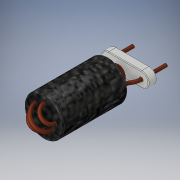
# Autodesk Inventor part: LairdTech_28C0236-0JW-10__
Saved by Autodesk Inventor 2019.1 (Build 231200000, 200)
## iProperties
Created: 2018-10-28
Part Number: LairdTech_28C0236-0JW-10__
Material: Generic
Document SubType Name: Modeling
Designer: huesof
Density: 1 g/cm^3
Appearance: Default
Author: huesof
Autodesk Inventor part; units mm, degrees
ref_plane "YZ Plane" through (0, 0, 0) normal (1, 0, 0) x (0, 1, 0)
ref_plane "XZ Plane" through (0, 0, 0) normal (0, 1, 0) x (-1, 0, 0)
ref_plane "XY Plane" through (0, 0, 0) normal (0, 0, 1) x (1, 0, 0)
sketch "Sketch1" plane through (0, 0, 0) normal (0, 0, 1) x (1, 0, 0)
  circle A0 centre (0, 0) radius 1.143
  circle A1 centre (5.08, 0) radius 1.143
  line L0 (0, 0) -> (0, 1.143) construction
  line L1 (5.08, 0) -> (5.08, 1.143) construction
  line L2 (0, 0) -> (0, -1.143) construction
  line L3 (5.08, 0) -> (5.08, -1.143) construction
  line L4 (0, 1.143) -> (5.08, 1.143)
  line L5 (5.08, -1.143) -> (0, -1.143)
  circle A2 centre (0, 0) radius 0.254
  circle A3 centre (5.08, 0) radius 0.254
  point P0 (1.7349, 0.2538)
  dimension "d0" = 2.286
  dimension "d1" = 2.286
  dimension "d2" = 0
  dimension "d3" = 5.08
  dimension "d4" = 0.508
  dimension "d5" = 0.508
  constraints: 12 end point, 5 coincident, 4 centre point, 4 point on circle, 2 point on line, 2 tangent, 1 parallel, 1 perpendicular
  measures "d0" diameter of A0
  measures "d1" diameter of A1
  measures "d2" vertical distance of point (0, 0) A1.centre
  measures "d3" distance of A1.centre point (0, 0)
  measures "d4" diameter of A2
  measures "d5" diameter of A3
extrude "Extrusion1" add sketch "Sketch1" along normal blind 1.27 contours A0 | A0 L4 A1 L5 | A1 | A2 | A3
hole "Hole1" at (5.08, 0, 0) at (0, 0, 0) direction (0, 0, 1) diameter 0.635 depth 1.27
extrude "Extrusion2" add sketch "Sketch1" along normal up to surface (1.27 mm away) separate body contours A2 | A3
extrude "Extrusion3" add sketch "Sketch1" against normal blind 5.08 contours A2 | A3 bodies 2
ref_plane "Work Plane1" through (0, 0, 3.81) normal (0, 0, 1) x (1, 0, 0)
sketch "Sketch2" plane through (0, 0, 3.81) normal (0, 0, 1) x (1, 0, 0)
  circle A0 centre (5.08, 0) radius 0.254 projected
  circle A1 centre (0, 0) radius 0.254 projected
  line L0 (0, 0) -> (5.08, 0) construction
  circle A2 centre (2.54, 0) radius 3
  circle A3 centre (2.54, 1.7526) radius 0.3175
  circle A4 centre (1.3007, 1.2393) radius 0.3175
  line L1 (2.54, 0) -> (1.3007, 1.2393) construction
  line L2 (2.54, 0) -> (4.2926, 0) construction
  circle A5 centre (0.7874, 0) radius 0.3175
  circle A6 centre (2.54, -1.7526) radius 0.3175
  circle A7 centre (3.7793, -1.2393) radius 0.3175
  circle A8 centre (4.2926, 0) radius 0.3175
  dimension "d20" = 6
  dimension "d24" = 0
  dimension "d26" = 1.7526
  dimension "d27" = 0.635
  dimension "d29" = 0.635
  dimension "d30" = 1.7526
  dimension "d31" = 225
  dimension "d36" = 0.635
  dimension "d37" = 1.7526
  dimension "d40" = 360
  constraints: 7 centre point, 6 end point, 2 coincident, 2 horizontal, 1 equal length, 1 midpoint, 1 point on line, 13 other
  measures "d20" diameter of A2
  measures "d24" horizontal distance of point (2.54, 0) A3.centre
  measures "d26" distance of point (2.54, 0) A3.centre
  measures "d27" diameter of A3
  measures "d29" diameter of A4
  measures "d30" distance of L1.start L1.end
  measures "d36" diameter of A5
  measures "d37" distance of point (2.54, 0) A5.centre
extrude "Extrusion4" add sketch "Sketch2" along normal blind 10 separate body contours A0 | A1 | A2
sketch "Sketch3" plane through (0, 0, 0) normal (0, 1, 0) x (-1, 0, 0)
  line L0 (-0.4699, 3.81) -> (-1.1049, 3.81) construction
  line L1 (-0.7874, 3.81) -> (0, 1.27) construction
  line L2 (-0.3175, 1.27) -> (0.3175, 1.27) construction
  line L3 (-5.3975, 1.27) -> (-4.7625, 1.27) construction
  line L4 (-5.08, 1.27) -> (-4.2926, 3.81) construction
  line L5 (-3.9751, 3.81) -> (-4.6101, 3.81) construction
  line L6 (0, 1.27) -> (-5.08, 1.27) construction
  arc A0 (-4.6863, 2.54) -> (-5.08, 1.27) centre (-2.5416, 1.1791) ccw
  line L7 (1.143, 1.27) -> (0, 1.27) projected
  arc A1 (0, 1.27) -> (-0.3937, 2.54) centre (-2.5384, 1.1791) ccw
  arc A2 (-0.7874, 3.81) -> (-0.3937, 2.54) centre (1.751, 3.9009) ccw
  arc A3 (-4.6863, 2.54) -> (-4.2926, 3.81) centre (-6.831, 3.9009) ccw
  point P0 (0, 0)
  dimension "d42" = 2.54
  dimension "d43" = 2.54
  dimension "d44" = 2.54
  dimension "d45" = 2.54
  constraints: 8 point on circle, 6 midpoint, 4 centre point, 4 end point, 2 point on line
  measures "d42" radius of A0
  measures "d43" radius of A1
  measures "d44" radius of A3
  measures "d45" radius of A2
sketch "Sketch4" plane through (5.08, 0, 1.27) normal (0, 0, 1) x (1, 0, 0)
  circle A0 centre (0, 0) radius 0.254 projected
  circle A1 centre (-5.08, 0) radius 0.254 projected
sweep "Sweep1" add profiles "Sketch4" path "Sketch3" bodies 2 path curves A0 A3 contours A0
sweep "Sweep2" add profiles "Sketch4" path "Sketch3" bodies 2 path curves A1 A2 contours A1
sketch "Sketch5" plane through (4.2926, 0, 3.81) normal (0, 0, 1) x (1, 0, 0)
  circle A0 centre (0, 0) radius 0.254 projected
  circle A1 centre (-3.5052, 0) radius 0.254 projected
  point P0 (-4.2926, 0)
  point P1 (0.254, 0)
  point P2 (-3.2512, 0)
  constraints: 2 horizontal alignment
extrude "Extrusion5" add sketch "Sketch5" along normal up to surface (10 mm away) bodies 2
sketch "Sketch6" plane through (0.7874, 0, 13.81) normal (0, 0, 1) x (1, 0, 0)
  circle A0 centre (0, 0) radius 0.254 projected
  circle A1 centre (3.5052, 0) radius 0.254 projected
  circle A2 centre (1.7526, 1.7526) radius 0.3175 projected
  circle A3 centre (0.5133, 1.2393) radius 0.3175 projected
  circle A4 centre (1.7526, -1.7526) radius 0.3175 projected
  circle A5 centre (2.9919, -1.2393) radius 0.3175 projected
  circle A6 centre (2.9919, -1.2393) radius 0.254
  line L0 (0, 0) -> (3.5052, 0) construction
  line L1 (1.7526, 0) -> (3.8739, 2.1213) construction
  line L2 (1.7526, 0) -> (4.7526, 0) construction
  circle A7 centre (1.7526, -1.7526) radius 0.254
  circle A8 centre (0.5133, 1.2393) radius 0.254
  circle A9 centre (1.7526, 1.7526) radius 0.254
  point P0 (-0.7874, 0)
  dimension "d52" = 0.508
  dimension "d53" = 0.508
  dimension "d54" = 3
  dimension "d55" = 45
  dimension "d57" = 0.508
  dimension "d59" = 0.508
  dimension "d61" = 0.508
  constraints: 6 end point, 4 centre point, 4 coincident, 2 horizontal, 1 equal length, 1 midpoint
  measures "d52" diameter of A6
  measures "d53" diameter of A1
  measures "d54" distance of L1.start L1.end
  measures "d55" angle of L2 L1
  measures "d57" diameter of A7
  measures "d59" diameter of A8
  measures "d61" diameter of A9
revolve "Revolution1" add sketch "Sketch6" angle 180 about axis through (2.54, 0, 13.81) along (-0.7071068, -0.7071068, 0) bodies 2 contours A1 | A6 | A7
extrude "Extrusion6" add sketch "Sketch6" against normal up to surface (10 mm away) contours A6 | A7 | A8 | A9 bodies 2
sketch "Sketch7" plane through (2.54, -1.7526, 3.81) normal (0, 0, -1) x (-1, 0, 0)
  circle A0 centre (0, 0) radius 0.254 projected
  circle A1 centre (-1.2393, 0.5133) radius 0.254 projected
  circle A2 centre (1.2393, 2.9919) radius 0.254 projected
  circle A3 centre (0, 3.5052) radius 0.254 projected
  circle A4 centre (-1.2393, 0.5133) radius 0.3175 construction
  line L0 (-1.2393, 0.5133) -> (1.2393, 2.9919) construction
  line L1 (0, 0) -> (0, 3.5052) construction
  line L2 (0, 1.7526) -> (-0.8423, 2.1015) construction
  line L3 (1.2393, 2.9919) -> (0, 3.5052) construction
  point P0 (2.54, 1.7526)
  constraints: 8 end point, 1 midpoint, 1 parallel, 1 vertical
revolve "Revolution2" add sketch "Sketch7" angle 180 about axis through (2.54, 0, 3.81) along (0.9238795, 0.3826834, 0) bodies 2 contours A0 | A1
fillet "Fillet1" radius 0.2 2 edges at (-0.46, 0, 13.81) (-0.46, 0, 3.81)
fillet "Fillet2" radius 0.1 8 edges at (-1.143, 0, 1.27) (2.54, -1.143, 1.27) (6.223, 0, 1.27) (2.54, 1.143, 1.27) (-1.143, 0, 0) (2.54, -1.143, 0) (6.223, 0, 0) (2.54, 1.143, 0)
thicken "Thicken1" operation add thickness 2.54 both sides no extend neighbours yes toward (0, 0, 1) bodies 2 faces at (-0.075, -0.0393, -5.08)
thicken "Thicken2" operation add thickness 2.54 both sides no extend neighbours yes toward (0, 0, 1) bodies 2 faces at (4.994, 0.084, -5.08)
equation "\"d1\" = d0"
equation "\"d5\" = d4"
equation "\"d29\" = d27"
equation "\"d30\" = d26"
equation "\"d36\" = d27"
equation "\"d37\" = d26"
equation "\"d43\" = d42"
equation "\"d44\" = d42"
equation "\"d45\" = d43"
equation "\"d52\" = d53"
equation "\"d57\" = d58"
equation "\"d59\" = d60"
equation "\"d61\" = d62"
equation "\"d58\" = 0.508"
equation "\"d60\" = 0.508"
equation "\"d62\" = 0.508"
body "Solid1"
body "Solid2"
body "Solid3"
